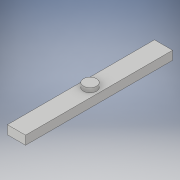
# Autodesk Inventor part: cam_mock
Saved by Autodesk Inventor 2019 (Build 230136000, 136)
## iProperties
Created: 2019-07-10
Part Number: cam_mock
Material: Generic
Document SubType Name: Modeling
Designer: Lino P
Density: 1 g/cm^3
Appearance: Default
Author: Lino P
Autodesk Inventor part; units mm, degrees
ref_plane "YZ Plane" through (0, 0, 0) normal (1, 0, 0) x (0, 1, 0)
ref_plane "XZ Plane" through (0, 0, 0) normal (0, 1, 0) x (-1, 0, 0)
ref_plane "XY Plane" through (0, 0, 0) normal (0, 0, 1) x (1, 0, 0)
sketch "Sketch1" plane through (0, 0, 0) normal (0, 1, 0) x (-1, 0, 0)
  line L0 (0, 0) -> (8.3, 0)
  line L1 (8.3, 0) -> (8.3, -67.4)
  line L2 (8.3, -67.4) -> (0, -67.4)
  line L3 (0, -67.4) -> (0, 0)
  dimension "d0" = 8.3
  dimension "d1" = 67.4
  constraints: 8 end point, 2 parallel, 1 horizontal, 1 perpendicular
  measures "d0" distance of L1.end L2.end
  measures "d1" distance of L0.end L1.end
extrude "Extrusion1" add sketch "Sketch1" along normal blind 4
sketch "Sketch2" plane through (0, 4, 0) normal (0, 1, 0) x (1, 0, 0)
  line L0 (-8.3, 0) -> (0, 0) construction
  line L1 (0, 0) -> (0, 67.4) construction
  line L2 (0, 67.4) -> (-8.3, 67.4) construction
  line L3 (-8.3, 67.4) -> (-8.3, 0) construction
  circle A0 centre (-4.15, 33.7) radius 3
  dimension "d4" = 6
  constraints: 1 centre point
  measures "d4" diameter of A0
extrude "Extrusion2" add sketch "Sketch2" along normal blind 2
body "Solid1"
